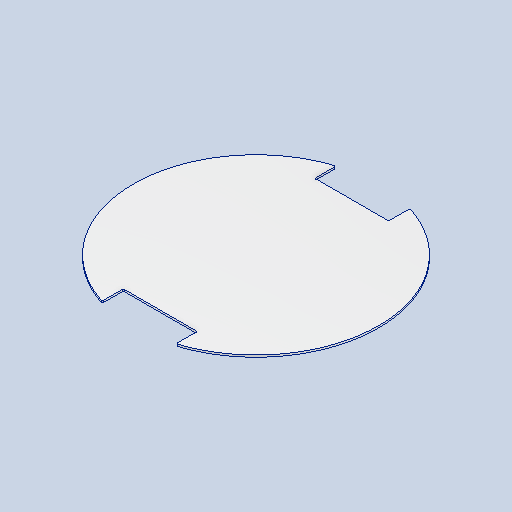
# Autodesk Inventor part: AMR_base
Saved by Autodesk Inventor 2026 (Build 300175050, 175E)
## iProperties
Created: 2025-11-23
Part Number: AMR_base
Material: Aluminum 6061
Document SubType Name: Modeling
Designer: Kartik
Mass: 1324.61 g
Surface Area: 2856.59 cm^2
Volume: 490.595 cm^3
Density: 2.7 g/cm^3
Appearance: Aluminum - Flat
Author: Kartik
Autodesk Inventor part; units mm, degrees
ref_plane "YZ Plane" through (0, 0, 0) normal (1, 0, 0) x (0, 1, 0)
ref_plane "XZ Plane" through (0, 0, 0) normal (0, 1, 0) x (-1, 0, 0)
ref_plane "XY Plane" through (0, 0, 0) normal (0, 0, 1) x (1, 0, 0)
sketch "Sketch1" plane through (0, 0, 0) normal (0, 1, 0) x (-1, 0, 0)
  circle A0 centre (0, 0) radius 220
  dimension "d0" = 440
  constraints: 1 centre point, 1 coincident
  measures "d0" diameter of A0
extrude "Extrusion1" add sketch "Sketch1" along normal blind 3.5
sketch "Sketch2" plane through (0, 3.5, 0) normal (0, 1, 0) x (1, 0, 0)
  line L0 (-66.25, 171.8) -> (66.25, 171.8)
  line L1 (66.25, 171.8) -> (66.25, 220)
  line L2 (66.25, 220) -> (-66.25, 220)
  line L3 (-66.25, 220) -> (-66.25, 171.8)
  circle A0 centre (0, 0) radius 220 projected
  point P0 (0, 220)
  dimension "d3" = 132.5
  dimension "d4" = 48.2
  dimension "d5" = 0
  dimension "d6" = 220
  constraints: 8 end point, 2 parallel, 1 horizontal, 1 midpoint, 1 perpendicular
  measures "d3" distance of L1.end L2.end
  measures "d4" distance of L0.end L1.end
  measures "d5" horizontal distance of point (0, 0) point (0, 220)
  measures "d6" distance of point (0, 220) point (0, 0)
extrude "Extrusion2" cut sketch "Sketch2" against normal through all contours L3 A0 L1 L0 | L3 L2 A0 | A0 L2 L1 picked at (0, 187.8667)
fillet "Fillet1" radius 2 4 edges at (-66.25, 1.75, -171.8) (-66.25, 1.75, -209.7878) (66.25, 1.75, -209.7878) (66.25, 1.75, -171.8)
mirror "Mirror1" about plane through (0, 0, 0) normal (0, 0, 1) of "Extrusion2", "Fillet1"
body "Solid1"
